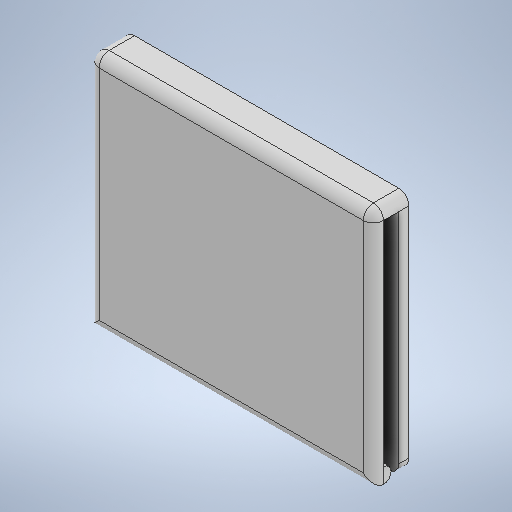
# Autodesk Inventor part: belt_clip
Saved by Autodesk Inventor 2025.2 (Build 292293000, 293)
## iProperties
Created: 2025-01-09
Part Number: belt_clip
Material: Generic
Document SubType Name: Modeling
Designer: tompe
Density: 1 g/cm^3
Appearance: Default
Author: tompe
Autodesk Inventor part; units mm, degrees
ref_plane "YZ Plane" through (0, 0, 0) normal (1, 0, 0) x (0, 1, 0)
ref_plane "XZ Plane" through (0, 0, 0) normal (0, 1, 0) x (-1, 0, 0)
ref_plane "XY Plane" through (0, 0, 0) normal (0, 0, 1) x (1, 0, 0)
sketch "Sketch1" plane through (0, 0, 0) normal (1, 0, 0) x (0, 1, 0)
  line L0 (0, 0) -> (0, -2)
  line L1 (0, -2) -> (45, -2)
  line L2 (45, -2) -> (45, -5)
  line L3 (45, -5) -> (0, -5)
  line L4 (0, 0) -> (47, 0)
  line L5 (47, 0) -> (47, -7)
  line L6 (47, -7) -> (0, -7)
  line L7 (0, -7) -> (0, -5)
  circle A0 centre (1.5, -2) radius 1.5
  point P0 (3, -2)
  point P1 (32, -2)
  point P2 (32, -5)
  dimension "d0" = 2
  dimension "d1" = 45
  dimension "d2" = 3
  dimension "d3" = 47
  dimension "d4" = 7
  dimension "d5" = 3
  dimension "d6" = 1.5
  constraints: 16 end point, 6 perpendicular, 2 point on line, 1 centre point, 1 horizontal, 1 vertical
  measures "d0" distance of L0.start L0.end
  measures "d1" distance of L0.end L1.end
  measures "d2" distance of L1.end L2.end
  measures "d3" distance of L0.start L4.end
  measures "d4" distance of L4.end L5.end
  measures "d5" diameter of A0
  measures "d6" distance of L0.end A0.centre
extrude "Extrusion1" add sketch "Sketch1" along normal blind 56
sketch "Sketch3" plane through (0, 0, 0) normal (0, 1, 0) x (-1, 0, 0)
  line L0 (0, -7) -> (-56, -7) projected
  line L1 (-34.7, -7) -> (-21.3, -7)
  line L2 (-21.3, -7) -> (-18.5, -9.8)
  line L3 (-18.5, -9.8) -> (-37.5, -9.8)
  line L4 (-34.7, -7) -> (-37.5, -9.8)
  line L5 (-56, -5) -> (-56, -7) projected
  point P0 (0, 0)
  point P1 (-28, -7)
  point P2 (-56, -6)
  point P3 (-21.3, -7)
  dimension "d10" = 135
  dimension "d11" = 135
  dimension "d12" = 2.8
  dimension "d13" = 28
  dimension "d14" = 19
  constraints: 8 end point, 3 midpoint, 1 horizontal, 1 parallel
  measures "d10" angle of L1 L2
  measures "d11" angle of L1 L4
  measures "d12" distance between parallel lines of L3 L1
  measures "d13" horizontal distance of point (-56, -6) point (-28, -7)
  measures "d14" distance of L2.end L3.end
extrude "Extrusion2" add sketch "Sketch3" along normal blind 30
fillet "Rundung1" radius 2 8 edges at (56, 47, -3.5) (56, 0, -6) (0, 47, -3.5) (0, 0, -6) (0, 23.5, 0) (28, 47, 0) (56, 23.5, 0) (28, 0, 0)
body "Solid1"
